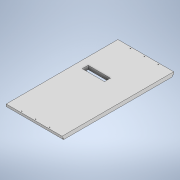
# Autodesk Inventor part: bench
Saved by Autodesk Inventor 2022 (Build 260153000, 153)
## iProperties
Created: 2022-02-20
Part Number: bench
Material: Generic
Document SubType Name: Modeling
Designer: MarkP
Density: 1 g/cm^3
Appearance: Default
Author: MarkP
Autodesk Inventor part; units mm, degrees
ref_plane "YZ Plane" through (0, 0, 0) normal (1, 0, 0) x (0, 1, 0)
ref_plane "XZ Plane" through (0, 0, 0) normal (0, 1, 0) x (-1, 0, 0)
ref_plane "XY Plane" through (0, 0, 0) normal (0, 0, 1) x (1, 0, 0)
sketch "Sketch1" plane through (0, 0, 0) normal (0, 1, 0) x (-1, 0, 0)
  line L0 (0, 0) -> (750, 0)
  line L1 (750, 0) -> (750, -1500)
  line L2 (750, -1500) -> (0, -1500)
  line L3 (0, -1500) -> (0, 0)
  line L4 (750, -1500) -> (750, -1480)
  line L5 (750, -1480) -> (0, -1480)
  line L6 (0, -1500) -> (750, -1500)
  line L7 (0, 0) -> (0, -20)
  line L8 (0, -20) -> (750, -20)
  line L9 (750, 0) -> (0, 0)
  dimension "d2" = 750
  dimension "d3" = 1500
  dimension "d6" = 20
  dimension "d7" = 20
  constraints: 20 end point, 4 equal length, 4 point on line, 3 perpendicular, 1 horizontal
  measures "d2" distance of L1.end L2.end
  measures "d3" distance of L0.end L1.end
  measures "d6" distance of L1.end L4.end
  measures "d7" distance of L0.start L7.end
extrude "Extrusion1" add sketch "Sketch1" along normal blind 50
sketch "Sketch2" plane through (0, 0, 0) normal (0, -1, 0) x (1, 0, 0)
  line L0 (0, 0) -> (0, -1500) projected
  line L1 (-750, -1500) -> (-750, 0) projected
  line L2 (0, 0) -> (-750, 0)
  line L3 (-750, 0) -> (-750, -20)
  line L4 (-750, -20) -> (0, -20)
  line L5 (0, -20) -> (0, 0)
  line L6 (0, -1500) -> (-750, -1500)
  line L7 (-750, -1500) -> (-750, -1480)
  line L8 (-750, -1480) -> (0, -1480)
  line L9 (0, -1480) -> (0, -1500)
  dimension "d8" = 20
  dimension "d9" = 20
  constraints: 16 end point, 4 parallel, 2 horizontal, 2 perpendicular, 2 point on line
  measures "d8" distance of L3.end L2.end
  measures "d9" distance of L6.end L7.end
extrude "Extrusion2" cut sketch "Sketch2" against normal blind 20 contours L0 L4 L1 L2 | L0 L6 L1 L8
sketch "Sketch3" plane through (0, 0, 0) normal (0, -1, 0) x (1, 0, 0)
  line L0 (0, -20) -> (0, -1480) projected
  circle A0 centre (-562, -20) radius 5
  circle A1 centre (-375, -20) radius 5
  circle A2 centre (-188, -20) radius 5
  line L1 (-750, -1480) -> (0, -1480) projected
  line L2 (-188, -20) -> (1272, -20) construction
  line L3 (-375, -20) -> (1085, -20) construction
  line L4 (0, -20) -> (-750, -20) projected
  line L5 (-562, -20) -> (898, -20) construction
  circle A3 centre (-562, -1480) radius 5
  circle A4 centre (-375, -1480) radius 5
  circle A5 centre (-188, -1480) radius 5
  point P0 (0, 0)
  dimension "d15" = 10
  dimension "d16" = 10
  dimension "d17" = 10
  dimension "d24" = 10
  dimension "d25" = 10
  dimension "d26" = 10
  constraints: 6 centre point, 6 end point, 3 horizontal
  measures "d15" diameter of A0
  measures "d16" diameter of A1
  measures "d17" diameter of A2
  measures "d24" diameter of A3
  measures "d25" diameter of A4
  measures "d26" diameter of A5
extrude "Extrusion3" cut sketch "Sketch3" against normal blind 61.275
thread "Thread1" size "M10x1.5" class "6H" standard "ANSI Metric M Profile" full length
thread "Thread2" size "M10x1.5" class "6H" standard "ANSI Metric M Profile" full length
thread "Thread3" size "M10x1.5" class "6H" standard "ANSI Metric M Profile" full length
thread "Thread4" size "M10x1.5" class "6H" standard "ANSI Metric M Profile" full length
thread "Thread5" size "M10x1.5" class "6H" standard "ANSI Metric M Profile" full length
thread "Thread6" size "M10x1.5" class "6H" standard "ANSI Metric M Profile" full length
sketch "Sketch4" plane through (0, 50, 0) normal (0, 1, 0) x (1, 0, 0)
  line L0 (-650, 1000) -> (-350, 1000)
  line L1 (-350, 1000) -> (-350, 920)
  line L2 (-350, 920) -> (-650, 920)
  line L3 (-650, 920) -> (-650, 1000)
  point P0 (0, 0)
  point P1 (-750, 1500)
  dimension "d47" = 300
  dimension "d48" = 80
  constraints: 8 end point, 2 parallel, 1 horizontal, 1 perpendicular
  measures "d47" distance of L1.end L2.end
  measures "d48" distance of L0.end L1.end
extrude "Extrusion4" cut sketch "Sketch4" against normal blind 220.025
body "Solid1"
